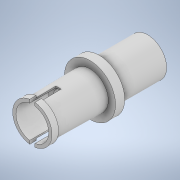
# Autodesk Inventor part: AxleGBR
Saved by Autodesk Inventor 2020.1 (Build 241239000, 239)
## iProperties
Created: 2020-03-14
Part Number: AxleGBR
Material: Generic
Document SubType Name: Modeling
Designer: super
Density: 1 g/cm^3
Appearance: Default
Author: super
Autodesk Inventor part; units mm, degrees
ref_plane "YZ Plane" through (0, 0, 0) normal (1, 0, 0) x (0, 1, 0)
ref_plane "XZ Plane" through (0, 0, 0) normal (0, 1, 0) x (-1, 0, 0)
ref_plane "XY Plane" through (0, 0, 0) normal (0, 0, 1) x (1, 0, 0)
sketch "Sketch1" plane through (0, 0, 0) normal (0, 1, 0) x (-1, 0, 0)
  line L0 (0, -1.778) -> (2.413, -1.778)
  line L1 (2.413, -1.778) -> (2.413, -10.16)
  line L2 (2.413, -10.16) -> (3.175, -10.16)
  line L3 (3.175, -10.16) -> (3.175, -11.43)
  line L4 (3.175, -11.43) -> (3.683, -11.43)
  line L5 (3.683, -11.43) -> (3.683, -2.032)
  line L6 (3.683, -2.032) -> (4.953, -2.032)
  line L7 (4.953, -2.032) -> (4.953, -0.254)
  line L8 (0, -0.254) -> (0, -1.778)
  line L9 (0, -0.254) -> (2.413, -0.254)
  line L10 (2.413, -0.254) -> (2.413, 4.572)
  line L11 (2.413, 4.572) -> (3.175, 4.572)
  line L12 (3.175, 4.572) -> (3.175, 10.922)
  line L13 (3.175, 10.922) -> (3.81, 10.922)
  line L14 (3.81, 10.922) -> (3.81, 9.652)
  line L15 (4.953, -0.254) -> (3.683, -0.254)
  line L16 (3.683, -0.254) -> (3.429, -0.254)
  line L17 (3.556, -0.254) -> (3.429, 9.652)
  line L18 (3.81, 9.652) -> (3.429, 9.652)
  line L19 (0, 10.922) -> (0, -12.4282) construction
  point P0 (0, 0)
  dimension "d0" = 1.778
  dimension "d1" = 2.413
  dimension "d2" = 8.382
  dimension "d3" = 0.762
  dimension "d4" = 1.27
  dimension "d5" = 0.508
  dimension "d6" = 9.398
  dimension "d7" = 1.27
  dimension "d8" = 1.778
  dimension "d9" = 4.826
  dimension "d10" = 0.762
  dimension "d11" = 6.35
  dimension "d12" = 0.635
  dimension "d13" = 1.27
  dimension "d14" = 1.27
  dimension "d15" = 0.254
  constraints: 40 end point, 9 perpendicular, 4 horizontal, 2 vertical, 1 midpoint, 1 parallel, 1 point on line
  measures "d0" distance of point (0, 0) L0.start
  measures "d1" distance of L0.start L0.end
  measures "d2" distance of L0.end L1.end
  measures "d3" distance of L1.end L2.end
  measures "d4" distance of L2.end L3.end
  measures "d5" distance of L3.end L4.end
  measures "d6" distance of L4.end L5.end
  measures "d7" distance of L5.end L6.end
  measures "d8" distance of L6.end L7.end
  measures "d9" distance of L9.end L10.end
  measures "d10" distance of L10.end L11.end
  measures "d11" distance of L11.end L12.end
  measures "d12" distance of L12.end L13.end
  measures "d13" distance of L13.end L14.end
  measures "d14" distance of L7.end L15.end
  measures "d15" distance of L15.end L16.end
revolve "Revolution1" add sketch "Sketch1" angle 360 about axis through (0, 0, 10.922) along (0, 0, -1)
sketch "Sketch2" plane through (0, 0, 10.922) normal (0, 0, 1) x (1, 0, 0)
  circle A0 centre (0, 0) radius 3.81 projected
  line L0 (0, 3.81) -> (0.508, 3.81)
  line L1 (0, 3.81) -> (0.508, 3.81) construction
  line L2 (0.508, 3.81) -> (0.508, 2.9079)
  line L3 (0.508, 2.9079) -> (-0.508, 2.9079)
  line L4 (-0.508, 2.9079) -> (-0.508, 3.81)
  line L5 (-0.508, 3.81) -> (0, 3.81)
  line L6 (-0.508, -2.9079) -> (0.508, -2.9079)
  line L7 (0.508, -2.9079) -> (0.508, -3.81)
  line L8 (-0.508, -3.81) -> (-0.508, -2.9079)
  line L9 (0.508, -3.81) -> (0, -3.81)
  point P0 (-0.508, -3.776)
  point P1 (0.508, -3.776)
  point P2 (0.508, 3.776)
  point P3 (-0.508, 3.776)
  dimension "d17" = 0.508
  dimension "d18" = 0
  dimension "d19" = 1.016
  dimension "d22" = 360
  constraints: 20 end point, 4 perpendicular, 3 horizontal, 1 collinear, 1 point on line, 21 other
  measures "d17" distance of L0.start L0.end
  measures "d18" distance between parallel lines of L0 L1
  measures "d19" distance of L2.end L3.end
extrude "Extrusion1" cut sketch "Sketch2" against normal blind 5.08 contours L2 L3 L4 A0 | A0 L8 L6 L7
body "Solid1"
